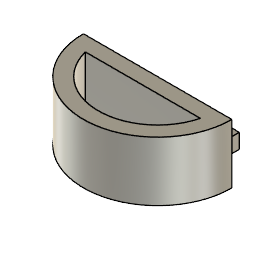
jellyfish v1 (Autodesk Fusion 360 design; units mm, degrees)
Autodesk Fusion 360 part; units mm, degrees
note: some values were not read from the file. Set by a fixed rule: which sketch regions a step uses.
sketch "Sketch1" plane through (0, 0, 0) normal (0, 0, 1) x (1, 0, 0)
  circle A0 centre (0, 0) radius 25
  line L0 (0, 0) -> (-25, 0)
  line L1 (0, 0) -> (25, 0)
  dimension "d1" = 50
  constraint coincident A0.centre L0.start
  constraint coincident A0 L0.end
  constraint horizontal L0
  constraint coincident A0 L1.end
  constraint parallel L0 L1
  measures "d1" diameter of A0
extrude "Extrude1" add sketch "Sketch1" along normal blind 20 contours A0 L0 L1 picked at (16.5736, -1.242)
sketch "Sketch2" plane through (0, 0, 0) normal (0, 1, 0) x (-1, 0, 0)
  line L0 (-25, 0) -> (25, 0)
  line L1 (25, 0) -> (25, 20)
  line L2 (25, 20) -> (-25, 20)
  line L3 (-25, 20) -> (-25, 0)
  line L4 (0, 0) -> (0, 20)
  line L5 (-25, 10) -> (25, 10)
  line L6 (0, 10) -> (-10, 10)
  line L7 (-10, 10) -> (-20, 10)
  line L8 (0, 10) -> (10, 10)
  line L9 (10, 10) -> (20, 10)
  line L10 (-17.5, 7.5) -> (-22.5, 7.5)
  line L11 (-22.5, 7.5) -> (-22.5, 12.5)
  line L12 (-22.5, 12.5) -> (-17.5, 12.5)
  line L13 (-17.5, 12.5) -> (-17.5, 7.5)
  line L14 (-17.5, 7.5) -> (-22.5, 12.5) construction
  line L15 (-22.5, 7.5) -> (-17.5, 12.5) construction
  line L16 (17.5, 12.5) -> (22.5, 12.5)
  line L17 (22.5, 12.5) -> (22.5, 7.5)
  line L18 (22.5, 7.5) -> (17.5, 7.5)
  line L19 (17.5, 7.5) -> (17.5, 12.5)
  line L20 (17.5, 12.5) -> (22.5, 7.5) construction
  line L21 (22.5, 12.5) -> (17.5, 7.5) construction
  line L22 (2.5, 7.5) -> (-2.5, 7.5)
  line L23 (-2.5, 7.5) -> (-2.5, 12.5)
  line L24 (-2.5, 12.5) -> (2.5, 12.5)
  line L25 (2.5, 12.5) -> (2.5, 7.5)
  line L26 (2.5, 7.5) -> (-2.5, 12.5) construction
  line L27 (-2.5, 7.5) -> (2.5, 12.5) construction
  point P0 (-20, 10)
  point P1 (20, 10)
  point P2 (0, 10)
  dimension "d4" = 10
  dimension "d5" = 10
  dimension "d6" = 10
  dimension "d7" = 10
  dimension "d8" = 5
  dimension "d9" = 5
  dimension "d10" = 5
  dimension "d11" = 5
  dimension "d12" = 5
  dimension "d13" = 5
  constraint coincident L4.start origin
  constraint midpoint L2 L4.end
  constraint midpoint L3 L5.start
  constraint midpoint L1 L5.end
  constraint midpoint L5 P2
  constraint perpendicular L4 L6
  constraint parallel L5 L7
  constraint perpendicular L4 L8
  constraint parallel L5 L9
  constraint horizontal L10
  constraint perpendicular L10 L11
  constraint parallel L10 L12
  constraint parallel L11 L13
  constraint coincident L14 P0
  constraint coincident L15 P0
  constraint coincident P0 L7.end
  constraint horizontal L16
  constraint perpendicular L16 L17
  constraint parallel L16 L18
  constraint parallel L17 L19
  constraint coincident L20 P1
  constraint coincident L21 P1
  constraint coincident P1 L9.end
  constraint horizontal L22
  constraint perpendicular L22 L23
  constraint parallel L22 L24
  constraint parallel L23 L25
  constraint coincident L26 P2
  constraint coincident L27 P2
  constraint coincident P2 L6.start
  measures "d4" distance of P2 L6.end
  measures "d5" distance of L6.end P0
  measures "d6" distance of P2 L8.end
  measures "d7" distance of L8.end P1
  measures "d8" distance of L10.end L11.end
  measures "d9" distance of L11.end L12.end
  measures "d10" distance of L16.end L17.end
  measures "d11" distance of L17.end L18.end
  measures "d12" distance of L22.end L23.end
  measures "d13" distance of L23.end L24.end
extrude "Extrude2" add sketch "Sketch2" along normal blind 5 contours L4 L5 L6 L22 L23 | L4 L5 L8 L22 L25 | L5 L7 L11 L12 L13 | L5 L7 L10 L11 L13 | L4 L5 L6 L23 L24 | L4 L5 L8 L24 L25 | L5 L9 L17 L18 L19 | L5 L9 L16 L17 L19
sketch "Sketch3" plane through (0, 0, 20) normal (0, 0, 1) x (-1, 0, 0)
  arc A0 (25, 0) -> (-25, 0) centre (0, 0) ccw
  line L0 (-25, 0) -> (25, 0)
  circle A1 centre (0, 0) radius 20
  line L1 (0, 0) -> (0, 5)
  line L2 (0, 5) -> (19.3649, 5)
  line L3 (0, 5) -> (-19.3649, 5)
  dimension "d16" = 40
  dimension "d17" = 5
  constraint concentric A0 A1
  constraint coincident A0.centre A1.centre
  constraint perpendicular L0 L1
  constraint coincident A1 L2.end
  constraint perpendicular L1 L2
  constraint coincident A1 L3.end
  constraint perpendicular L1 L3
  measures "d16" diameter of A1
  measures "d17" distance of A0.centre L1.end
extrude "Extrude3" cut sketch "Sketch3" against normal blind 20 contours A1 L2 L3
sketch "Sketch4" plane through (0, 0, 12.5) normal (0, 0, 1) x (-1, 0, 0)
  line L0 (-17.5, 0) -> (-22.5, 0)
  line L1 (-22.5, 0) -> (-22.5, -5)
  line L2 (-22.5, -5) -> (-17.5, -5)
  line L3 (-17.5, -5) -> (-17.5, 0)
  circle A0 centre (-20, -2.5) radius 1
  dimension "d20" = 2
  measures "d20" diameter of A0
extrude "Extrude4" add sketch "Sketch4" along normal blind 3 contours A0
sketch "Sketch5" plane through (0, 0, 12.5) normal (0, 0, 1) x (-1, 0, 0)
  line L0 (2.5, 0) -> (-2.5, 0)
  line L1 (-2.5, 0) -> (-2.5, -5)
  line L2 (-2.5, -5) -> (2.5, -5)
  line L3 (2.5, -5) -> (2.5, 0)
  line L4 (0, -5) -> (0, 0)
  circle A0 centre (0, -2.5) radius 1
  dimension "d23" = 2
  constraint midpoint L2 L4.start
  constraint coincident L4.end origin
  constraint midpoint L4 A0.centre
  measures "d23" diameter of A0
extrude "Extrude5" add sketch "Sketch5" along normal blind 3 contours L4 A0 | L4 A0
sketch "Sketch6" plane through (0, 0, 12.5) normal (0, 0, 1) x (-1, 0, 0)
  line L0 (22.5, 0) -> (17.5, 0)
  line L1 (17.5, 0) -> (17.5, -5)
  line L2 (17.5, -5) -> (22.5, -5)
  line L3 (22.5, -5) -> (22.5, 0)
  line L4 (20, -5) -> (20, 0)
  circle A0 centre (20, -2.5) radius 1
  dimension "d26" = 2
  constraint midpoint L2 L4.start
  constraint midpoint L0 L4.end
  constraint midpoint L4 A0.centre
  measures "d26" diameter of A0
extrude "Extrude6" add sketch "Sketch6" along normal blind 3 contours L4 A0 | L4 A0
